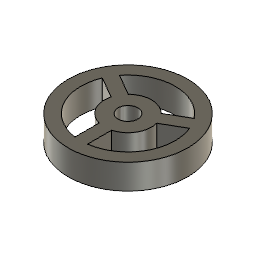
lighter_converyor_wheel (Autodesk Fusion 360 design; units mm, degrees)
Autodesk Fusion 360 part; units mm, degrees
sketch "Sketch1" plane through (0, 0, 0) normal (0, 0, 1) x (1, 0, 0)
  circle A0 centre (0, 0) radius 3.125
  circle A1 centre (0, 0) radius 19
  circle A2 centre (0, 0) radius 7.5
  circle A3 centre (0, 0) radius 15
  line L0 (-2, -6) -> (2, -6)
  line L1 (2, -6) -> (2, -16)
  line L2 (2, -16) -> (-2, -16)
  line L3 (-2, -16) -> (-2, -6)
  line L4 (4.1962, 4.7321) -> (12.8564, 9.7321)
  line L5 (14.8564, 6.2679) -> (6.1962, 1.2679)
  line L6 (-6.1962, 1.2679) -> (-14.8564, 6.2679)
  line L7 (-12.8564, 9.7321) -> (-4.1962, 4.7321)
  dimension "d1" = 6.25
  dimension "d2" = 38
  dimension "d3" = 15
  dimension "d5" = 360
  constraint coincident A0.centre A1.centre
  constraint concentric A0 A1
  constraint concentric A0 A2
  constraint concentric A2 A3
  constraint horizontal L0
  constraint vertical L1
  constraint horizontal L2
  constraint vertical L3
  measures "d1" diameter of A0
  measures "d2" diameter of A1
  measures "d3" diameter of A2
extrude "Extrude1" add sketch "Sketch1" along normal blind 8 contours A1 | A2 L0 L1 L3 | A2 A3 L4 L5 | A2 A3 L1 L3 | A2 L0 L1 L3 | A3 L1 L2 L3 | A2 A3 L6 L7
